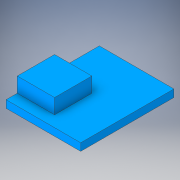
# Autodesk Inventor part: POWER_DELIVERY
Saved by Autodesk Inventor 2019 (Build 230136000, 136)
## iProperties
Created: 2020-03-13
Part Number: POWER_DELIVERY
Material: Generic
Document SubType Name: Modeling
Designer: Pulag
Density: 1 g/cm^3
Appearance: Default
Author: Pulag
Autodesk Inventor part; units mm, degrees
ref_plane "YZ Plane" through (0, 0, 0) normal (1, 0, 0) x (0, 1, 0)
ref_plane "XZ Plane" through (0, 0, 0) normal (0, 1, 0) x (-1, 0, 0)
ref_plane "XY Plane" through (0, 0, 0) normal (0, 0, 1) x (1, 0, 0)
sketch "Sketch1" plane through (0, 0, 0) normal (0, 1, 0) x (-1, 0, 0)
  line L0 (-10, 12.5) -> (10, 12.5)
  line L1 (10, 12.5) -> (10, -12.5)
  line L2 (10, -12.5) -> (-10, -12.5)
  line L3 (-10, -12.5) -> (-10, 12.5)
  line L4 (-10, 12.5) -> (10, -12.5) construction
  line L5 (10, 12.5) -> (-10, -12.5) construction
  point P0 (0, 0)
  dimension "d0" = 20
  dimension "d1" = 25
  constraints: 12 end point, 2 midpoint, 2 parallel, 1 horizontal, 1 perpendicular
  measures "d0" distance of L1.end L2.end
  measures "d1" distance of L0.end L1.end
extrude "Extrusion1" add sketch "Sketch1" along normal blind 2
sketch "Sketch2" plane through (0, 2, 0) normal (0, 1, 0) x (1, 0, 0)
  line L0 (-10, -9.5) -> (0, -9.5)
  line L1 (0, -9.5) -> (0, 0.5)
  line L2 (0, 0.5) -> (-10, 0.5)
  line L3 (-10, 0.5) -> (-10, -9.5)
  point P0 (0, 0)
  dimension "d4" = 10
  dimension "d5" = 10
  constraints: 8 end point, 2 parallel, 1 horizontal, 1 perpendicular
  measures "d4" distance of L2.end L1.end
  measures "d5" distance of L1.end L0.end
extrude "Extrusion2" add sketch "Sketch2" along normal blind 4
body "Solid1"
